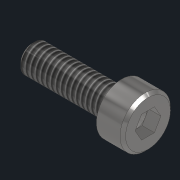
# Autodesk Inventor part: M2.5
Saved by Autodesk Inventor 2022 (Build 260153000, 153)
## iProperties
Part Number: M2.5
Material: 鋼、炭素鋼
Catalog Web Link: www.cadenas.de
Description: Screw1-Couplings - Hexagon Socket Head Cap Screw
Vendor: MISUMI
Document SubType Name: Modeling
Designer: partserver
Manufacturer: MISUMI
Mass: 0.563205 g
Surface Area: 1.32762 cm^2
Volume: 0.0717458 cm^3
Density: 7.85 g/cm^3
Appearance: 半つや出し
Category: PARTsolutions
Company: MISUMI
PSOL_IDENT_0: {$CADENAS_DATA\23d-libs\misumi\metric\50_couplings\parts\screw.prj},148 {VTYP=3D},{NB=M2.5},{LINA=M2
PSOL_IDENT_1: .5},{NN=Screw1},{DATE=30.06.2021 13:25:10},{GEOMDATE=15.07.2011 02:04:00},{VERSION=},{LINEID=20},{WB
PSOL_IDENT_2: VAR=},{WBNUMERIC=}  {NB=M2.5},{LINA=M2.5},{KT=DUMMY},{PN=M2.5},{THREAD=M2.5},{THMD1=2.5000},{THMIN1=
PSOL_IDENT_3: 2.0130},{KK=2.36},{L=8},{DK=4.5},{S=2.00},{TT=1.1},{EE=2.30},{DA=3.1},{DS=2.5},{VV=0.25},{RR=0.10}
NB: M2.5
NN: Screw1
NT: Couplings - Hexagon Socket Head Cap Screw
NBSYN: $PN.
LINA: M2.5
CATALOG: Misumi
PN: M2.5
KK: 2.36
L: 8
DK: 4.5
S: 2
TT: 1.1
EE: 2.3
DA: 3.1
DS: 2.5
VV: 0.25
RR: 0.1
SUPPLIER: MISUMI
ARTICLENO: M2.5
BOMINFO: M2.5
CREATOR: CADENAS GmbH
Title: M2.5
Author: Cadenas PARTsolutions
Comments: Couplings - Hexagon Socket Head Cap Screw
Autodesk Inventor part; units mm, degrees
sketch "Sketch_1" plane through (0, 0, 0) normal (0, 0, 1) x (1, 0, 0)
  line L0 (8, 0) -> (-2.36, 0)
  line L1 (-2.36, 0) -> (-2.36, 2)
  line L2 (-2.36, 2) -> (-2.11, 2.25)
  line L3 (-2.11, 2.25) -> (0, 2.25)
  line L4 (0, 2.25) -> (0, 1.25)
  line L5 (0, 1.25) -> (7.7565, 1.25)
  line L6 (7.7565, 1.25) -> (8, 1.0065)
  line L7 (8, 1.0065) -> (8, 0)
  line L8 (8, 0) -> (-2.36, 0)
  constraints: 18 end point
revolve "Revolution1" add sketch "Sketch_1" angle 360 about axis through (8, 0, 0) along (1, 0, 0)
thread "Thread1" size "M2.5x0.45" class "6g" standard "ISO Metric profile" length 7.2348
sketch "Sketch_2" plane through (-2.36, 0, 0) normal (1, 0, 0) x (0, 0, -1)
  line L0 (-1, -0.5774) -> (0, -1.1547)
  line L1 (0, -1.1547) -> (1, -0.5774)
  line L2 (1, -0.5774) -> (1, 0.5774)
  line L3 (1, 0.5774) -> (0, 1.1547)
  line L4 (0, 1.1547) -> (-1, 0.5774)
  line L5 (-1, 0.5774) -> (-1, -0.5774)
  constraints: 12 end point
extrude "Extrusion1" cut sketch "Sketch_2" along normal blind 1.1
sketch "Sketch_5" plane through (0, 0, 0) normal (0, 0, 1) x (1, 0, 0)
  line L0 (-0.6826, 0) -> (-1.26, 0)
  line L1 (-1.26, 0) -> (-1.26, 1)
  line L2 (-1.26, 1) -> (-0.6826, 0)
  line L3 (-0.6826, 0) -> (-1.26, 0)
  constraints: 8 end point
revolve "Revolution2" cut sketch "Sketch_5" angle 360 about axis through (-0.6826, 0, 0) along (1, 0, 0)
ref_plane "SCW_XY" through (0, 0, 0) normal (1, 0, 0) x (0, 0, -1)
ref_plane "SCW_YZ" through (0, 0, 0) normal (0, 0, -1) x (0, 1, 0)
ref_plane "SCW_ZX" through (0, 0, 0) normal (0, 1, 0) x (1, 0, 0)
body "Solid1"
